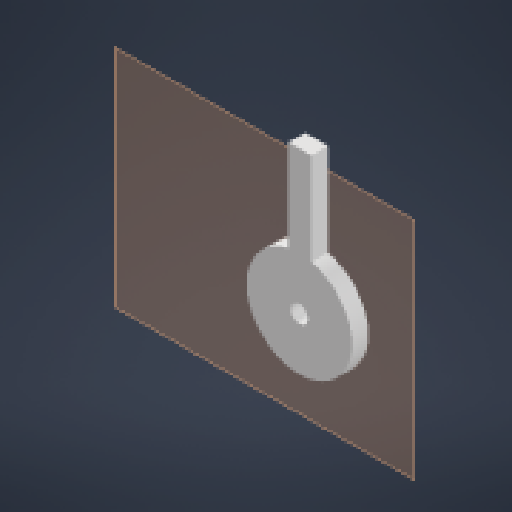
# Autodesk Inventor part: Driver
Saved by Autodesk Inventor 2023 (Build 270158000, 158)
## iProperties
Created: 2022-11-05
Part Number: Driver
Material: Generic
Document SubType Name: Modeling
Designer: cmzgt
Density: 1 g/cm^3
Appearance: Default
Author: cmzgt
Autodesk Inventor part; units mm, degrees
ref_plane "YZ Plane" through (0, 0, 0) normal (1, 0, 0) x (0, 1, 0)
ref_plane "XZ Plane" through (0, 0, 0) normal (0, 1, 0) x (-1, 0, 0)
ref_plane "Work Plane1" through (0, 0, 0) normal (0, 0, 1) x (1, 0, 0)
sketch "Sketch1" plane through (0, 0, 0) normal (0, 0, 1) x (1, 0, 0)
  circle A0 centre (52.5272, 25.8826) radius 2.413 projected
  circle A1 centre (52.5272, 25.8826) radius 0.8255 projected
  circle A2 centre (52.5272, 25.8826) radius 14.6558
  circle A3 centre (23.2156, 25.8826) radius 2.413 projected
  line L0 (52.7126, 40.5372) -> (52.7126, 65.9372)
  line L1 (52.7126, 40.5372) -> (78.1126, 40.5372) construction
  line L2 (52.7126, 65.9372) -> (55.8876, 65.9372)
  line L3 (55.8876, 65.9372) -> (55.8876, 40.148)
  line L4 (52.7126, 65.9372) -> (49.5376, 65.9372)
  line L5 (49.5376, 65.9372) -> (49.5376, 40.2302)
  point P0 (0, 0)
  dimension "d0" = 29.3116
  dimension "d2" = 25.4
  dimension "d3" = 90
  dimension "d4" = 3.175
  dimension "d5" = 0
  dimension "d6" = 3.175
  dimension "d7" = 14.6546
  constraints: 12 end point, 3 horizontal, 3 point on circle, 2 perpendicular, 1 centre point, 1 coincident, 1 vertical
  measures "d0" diameter of A2
  measures "d2" distance of L0.start L0.end
  measures "d3" angle of L1 L0
  measures "d4" distance of L0.end L2.end
  measures "d5" angle of L0 L3
  measures "d6" distance of L0.end L4.end
  measures "d7" distance from line of A1.centre L1
ref_plane "Work Plane2" through (20.8026, 23.4696, 4.6228) normal (0, 0, 1) x (1, 0, 0)
extrude "Extrusion1" add sketch "Sketch1" along normal up to surface (4.6228 mm away) contours A2 | A2 L0 L2 L3 | L5 L4 L0 A2
body "Solid1"
